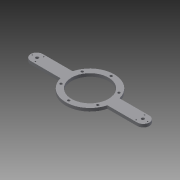
# Autodesk Inventor part: middle plate
Saved by Autodesk Inventor 2015 (Build 190159000, 159)
## iProperties
Created: 2015-02-28
Part Number: middle plate
Material: Generic
Document SubType Name: Modeling
Designer: Qiuyang
Density: 1 g/cm^3
Appearance: Default
Author: Qiuyang
Autodesk Inventor part; units mm, degrees
ref_plane "YZ Plane" through (0, 0, 0) normal (1, 0, 0) x (0, 1, 0)
ref_plane "XZ Plane" through (0, 0, 0) normal (0, 1, 0) x (-1, 0, 0)
ref_plane "XY Plane" through (0, 0, 0) normal (0, 0, 1) x (1, 0, 0)
sketch "Sketch4" plane through (0, 0, 0) normal (0, 1, 0) x (-1, 0, 0)
  circle A0 centre (0, 0) radius 38.735
  circle A1 centre (0, 0) radius 50.8
  dimension "d9" = 77.47
  dimension "d10" = 101.6
  constraints: 2 centre point, 2 coincident
  measures "d9" diameter of A0
  measures "d10" diameter of A1
extrude "Extrusion2" add sketch "Sketch4" along normal blind 6.35
sketch "Sketch5" plane through (0, 6.35, 0) normal (0, 1, 0) x (1, 0, 0)
  circle A0 centre (0, -44.45) radius 2.667
  circle A1 centre (38.4948, -22.225) radius 2.667
  circle A2 centre (38.4948, 22.225) radius 2.667
  circle A3 centre (0, 44.45) radius 2.667
  circle A4 centre (-38.4948, 22.225) radius 2.667
  circle A5 centre (-38.4948, -22.225) radius 2.667
  point P0 (0, 0)
  dimension "d13" = 5.334
  dimension "d16" = 360
  constraints: 6 centre point, 13 other
  measures "d13" diameter of A0
extrude "Extrusion3" cut sketch "Sketch5" against normal blind 6.35
sketch "Sketch7" plane through (0, 6.35, 0) normal (0, 1, 0) x (1, 0, 0)
  line L0 (-50.8, 12.7) -> (-111.76, 12.7)
  line L1 (-111.76, 12.7) -> (-111.76, -12.7)
  line L2 (-111.76, -12.7) -> (-50.8, -12.7)
  line L3 (-50.8, -12.7) -> (-50.8, 12.7)
  line L4 (50.8, 12.7) -> (111.76, 12.7)
  line L5 (111.76, 12.7) -> (111.76, -12.7)
  line L6 (111.76, -12.7) -> (50.8, -12.7)
  line L7 (50.8, -12.7) -> (50.8, 12.7)
  point P0 (0, 0)
  dimension "d46" = 60.96
  dimension "d47" = 25.4
  dimension "d48" = 60.96
  dimension "d49" = 25.4
  constraints: 16 end point, 4 parallel, 2 horizontal, 2 perpendicular
  measures "d46" distance of L2.end L1.end
  measures "d47" distance of L1.end L0.end
  measures "d48" distance of L5.end L6.end
  measures "d49" distance of L4.end L5.end
extrude "Extrusion4" add sketch "Sketch7" against normal blind 6.35
sketch "Sketch8" plane through (0, 6.35, 0) normal (0, 1, 0) x (1, 0, 0)
  line L0 (-123.5202, 12.7) -> (-50.8, 12.7) projected
  line L1 (-60.9386, 12.7) -> (-45.3133, 12.7)
  line L2 (-45.3133, 12.7) -> (-45.3133, -12.7)
  line L3 (-45.3133, -12.7) -> (-60.9386, -12.7)
  line L4 (-60.9386, -12.7) -> (-60.9386, 12.7)
  line L5 (57.1886, 12.7) -> (43.7508, 12.7)
  line L6 (43.7508, 12.7) -> (43.7508, -12.7)
  line L7 (43.7508, -12.7) -> (57.1886, -12.7)
  line L8 (57.1886, -12.7) -> (57.1886, 12.7)
  point P0 (0, 0)
  constraints: 16 end point, 4 parallel, 3 point on line, 2 horizontal, 2 perpendicular
extrude "Extrusion5" add sketch "Sketch8" against normal blind 6.35
sketch "Sketch9" plane through (0, 6.35, 0) normal (0, 1, 0) x (1, 0, 0)
  circle A0 centre (-111.7602, 0) radius 12.7
  line L0 (111.76, 12.7) -> (111.76, -12.7) projected
  circle A1 centre (111.76, 0) radius 12.7
  point P0 (0, 0)
  point P1 (-111.76, -12.7)
  constraints: 1 coincident, 1 midpoint, 1 vertical alignment, 5 other
extrude "Extrusion6" add sketch "Sketch9" against normal blind 6.35
sketch "Sketch10" plane through (0, 6.35, 0) normal (0, 1, 0) x (1, 0, 0)
  circle A0 centre (-110.8202, 0) radius 3.175
  circle A1 centre (110.8202, 0) radius 3.175
  circle A2 centre (120.904, 0) radius 1.27
  circle A3 centre (105.7783, 8.7328) radius 1.27
  circle A4 centre (105.7783, -8.7328) radius 1.27
  circle A5 centre (-120.904, 0) radius 1.27
  circle A6 centre (-105.7783, -8.7328) radius 1.27
  circle A7 centre (-105.7783, 8.7328) radius 1.27
  point P0 (0, 0)
  dimension "d32" = 6.35
  dimension "d33" = 6.35
  dimension "d34" = 2.54
  dimension "d37" = 360
  dimension "d39" = 2.54
  dimension "d42" = 360
  constraints: 8 centre point, 14 other
  measures "d32" diameter of A0
  measures "d33" diameter of A1
  measures "d34" diameter of A2
  measures "d39" diameter of A5
extrude "Extrusion7" cut sketch "Sketch10" against normal blind 6.35
body "Solid2"
